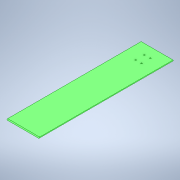
# Autodesk Inventor part: 前カバー中盤
Saved by Autodesk Inventor 2022 (Build 260153000, 153)
## iProperties
Created: 2022-11-07
Part Number: 前カバー中盤
Material: フェノール樹脂
Document SubType Name: Modeling
Designer: tdn82
Density: 1.38 g/cm^3
Appearance: 滑らか - 淡いオレンジ
Author: tdn82
Autodesk Inventor part; units mm, degrees
ref_plane "YZ Plane" through (0, 0, 0) normal (1, 0, 0) x (0, 1, 0)
ref_plane "XZ Plane" through (0, 0, 0) normal (0, 1, 0) x (-1, 0, 0)
ref_plane "XY Plane" through (0, 0, 0) normal (0, 0, 1) x (1, 0, 0)
sketch "スケッチ1" plane through (0, 0, 0) normal (0, 1, 0) x (-1, 0, 0)
  line L0 (0, 0) -> (-80, 0)
  line L1 (-80, 0) -> (-80, -336)
  line L2 (-80, -336) -> (0, -336)
  line L3 (0, -336) -> (0, 0)
  dimension "d0" = 336
  dimension "d1" = 80
  constraints: 8 end point, 2 parallel, 1 horizontal, 1 perpendicular
  measures "d0" distance of L2.end L0.start
  measures "d1" distance of L0.start L0.end
extrude "押し出し1" add sketch "スケッチ1" along normal blind 2
sketch "スケッチ3" plane through (0, 0, 0) normal (0, -1, 0) x (1, 0, 0)
  line L0 (80, -336) -> (0, -336) projected
  line L1 (80, 0) -> (80, -336) projected
  point P0 (0, 0)
  point P1 (48, -311)
  point P2 (33, -311)
  point P3 (48, -289)
  point P4 (33, -289)
  dimension "d20" = 25
  dimension "d21" = 32
  dimension "d24" = 15
  dimension "d27" = 22
  constraints: 1 horizontal, 1 vertical, 3 other
  measures "d20" distance from line of L0 point (48, -311)
  measures "d21" distance from line of point (48, -311) L1
  measures "d24" distance of point (48, -311) point (33, -311)
  measures "d27" distance of point (48, -311) point (48, -289)
hole "穴1" at (48, 0, -311) at (33, 0, -311) at (48, 0, -289) at (33, 0, -289) direction (0, 1, 0) diameter 3.2 end through all
chamfer "面取り2" distance 2 angle 45 1 edges at (40, 2, 0)
